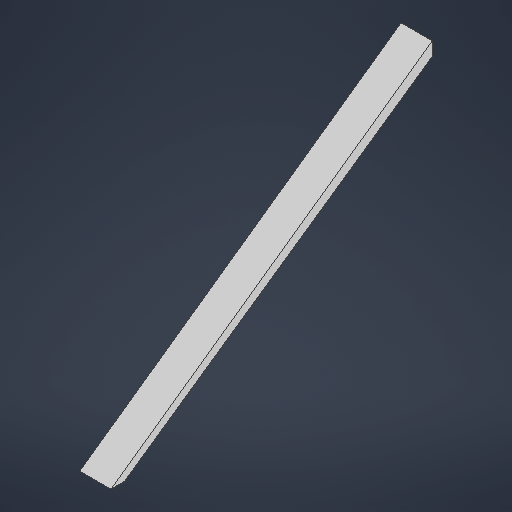
# Autodesk Inventor part: S_2x4x44.12
Saved by Autodesk Inventor 2027.1 (Build 311270010, 270A)
## iProperties
Created: 2026-08-30
Part Number: S_2x4x44.12
Material: Generic
Document SubType Name: Modeling
Designer: jorda
Density: 1 g/cm^3
Appearance: Default
Author: jorda
Autodesk Inventor part; units mm, degrees
ref_plane "YZ Plane" through (0, 0, 0) normal (1, 0, 0) x (0, 1, 0)
ref_plane "XZ Plane" through (0, 0, 0) normal (0, 1, 0) x (-1, 0, 0)
ref_plane "XY Plane" through (0, 0, 0) normal (0, 0, 1) x (1, 0, 0)
sketch "Sketch1" plane through (0, 0, 0) normal (1, 0, 0) x (0, 1, 0)
  line L0 (647.7, -914.4) -> (609.6, -914.4)
  line L1 (0, 0) -> (0, -38.1)
  line L2 (0, -38.1) -> (609.6, -914.4)
  line L3 (647.7, -914.4) -> (0, 0)
  constraints: 8 end point
extrude "Extrusion1" add sketch "Sketch1" along normal blind 88.9
body "Solid1"
